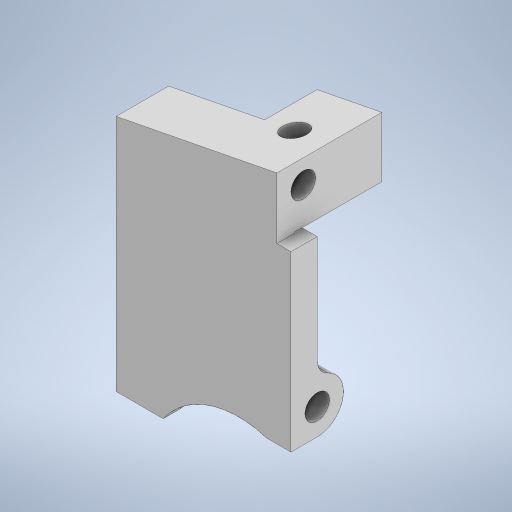
# Autodesk Inventor part: scianka_prawa
Saved by Autodesk Inventor 2023.5 (Build 275446000, 446)
## iProperties
Created: 2025-03-26
Part Number: scianka_prawa
Material: Ogólny
Document SubType Name: Modeling
Designer: kamil
Density: 1 g/cm^3
Appearance: Domyślna
Author: kamil
Autodesk Inventor part; units mm, degrees
ref_plane "YZ Plane" through (0, 0, 0) normal (1, 0, 0) x (0, 1, 0)
ref_plane "XZ Plane" through (0, 0, 0) normal (0, 1, 0) x (-1, 0, 0)
ref_plane "XY Plane" through (0, 0, 0) normal (0, 0, 1) x (1, 0, 0)
sketch "Szkic1" plane through (0, 0, 0) normal (0, 0, 1) x (1, 0, 0)
  line L0 (-34.4275, 20.8419) -> (2, 27.9622) projected
  line L1 (-2, 0) -> (-2, 27.1803) projected
  arc A0 (-16.6168, -4) -> (-14.1644, -18.5) centre (-8, -10) ccw projected
  circle A1 centre (-8, -10) radius 10.5
  line L2 (-2, 0) -> (-4.7984, 0)
  line L3 (-16.6168, -4) -> (-22, -4) projected
  line L4 (-22, 22.4466) -> (-22, 0.5) projected
  line L5 (-22, -4) -> (-22, 0.5)
  line L6 (-22, 22.4466) -> (-22, 23.271)
  point P0 (0, 0)
  constraints: 6 end point, 2 vertical, 1 coincident, 1 horizontal, 1 point on line, 4 other
extrude "Wyciągnięcie proste1" add sketch "Szkic1" against normal blind 2 contours L0 L1 L2 A1 L3 L5 L4 L6
sketch "Szkic2" plane through (-22, -4, 0) normal (-1, 0, 0) x (0, 0, 1)
  circle A0 centre (-2.5, 5.5) radius 1.3 projected
  line L0 (0, 27.271) -> (0, 0) projected
  circle A1 centre (-2.5, 5.5) radius 2.5
  line L1 (0, 27.271) -> (0, 0) projected
  line L2 (0, 27.271) -> (-2, 27.271) projected
  line L3 (-2, 0) -> (-2, 27.271) projected
  line L4 (0, 0) -> (-2, 0) projected
  line L5 (-2, 0) -> (-4.6176, 4.1711)
  line L6 (-2, 0) -> (-2, 27.271) projected
  line L7 (-2, 11) -> (-4.6176, 6.8289)
  point P0 (0, 4)
  constraints: 4 end point, 3 tangent, 2 point on circle, 1 centre point, 1 coincident, 1 point on line, 1 vertical alignment
extrude "Wyciągnięcie proste2" add sketch "Szkic2" against normal blind 5 contours L3 A0 | A0 L3 A1 | A1 L7 L3 | L3 L5 A1 picked at (-2.9631, 5.7248) picked at (-2.3031, 3.4223)
sketch "Szkic3" plane through (0, 0, -2) normal (0, 0, -1) x (-1, 0, 0)
  line L0 (2.5, 6.5) -> (19.5, 6.5) projected
  line L1 (2.5, 19.5) -> (2.5, 6.5) projected
  line L2 (19.5, 19.5) -> (2.5, 19.5) projected
  line L3 (19.5, 6.5) -> (19.5, 19.5) projected
  line L4 (2.5, 20) -> (19.5, 20) projected
  line L5 (17, 7) -> (22, 7) projected
  line L6 (22, 7) -> (22, 23.271) projected
  line L7 (22, 23.271) -> (2, 27.1803) projected
  line L8 (2, 27.1803) -> (2, 0) projected
  line L9 (2, 0) -> (4.7984, 0) projected
  arc A0 (16.6168, -4) -> (4.7984, 0) centre (8, -10) ccw projected
  line L10 (16.6168, -4) -> (17, -4) projected
  line L11 (17, -4) -> (17, 7) projected
  line L12 (19.5, 20) -> (22, 20)
  line L13 (22, 7) -> (22, 23.271) projected
  line L14 (2.5, 20) -> (2, 20)
  line L15 (2, 0) -> (2, 27.1803) projected
  point P0 (0, 0)
  constraints: 4 end point, 3 point on line, 1 perpendicular
extrude "Wyciągnięcie proste3" add sketch "Szkic3" along normal blind 4 contours L12 L4 L14 L8 L7 L6
sketch "Szkic4" plane through (0, 0, -6) normal (0, 0, -1) x (-1, 0, 0)
  line L0 (2, 20) -> (22, 20) projected
  line L1 (22, 20) -> (22, 23.271) projected
  line L2 (22, 23.271) -> (2, 27.1803) projected
  line L3 (2, 27.1803) -> (2, 20) projected
  line L4 (12.0145, 25.2228) -> (12.0145, 21) projected
  line L5 (12.0145, 21) -> (12, 20)
  line L6 (22, 20) -> (2, 20) projected
  point P0 (0, 0)
  constraints: 2 end point, 1 midpoint
extrude "Wyciągnięcie proste4" add sketch "Szkic4" along normal blind 6 contours L3 L2 L4 L5 L0
sketch "Szkic5" plane through (-12.0145, 21, -6) normal (-1, 0, 0) x (0, 0, 1)
  line L0 (0, 4.2228) -> (0, 0) projected
  line L1 (0, 4.2228) -> (-6, 4.2228) projected
  line L2 (-6, 0) -> (-6, 4.2228) projected
  line L3 (0, 0) -> (-6, 0) projected
  line L4 (0, 0) -> (-6, 0) projected
  line L5 (0, 0) -> (0, -1) projected
  line L6 (0, 0) -> (-6, 0) projected
  line L7 (-6, -1) -> (-6, 0) projected
  line L8 (0, -1) -> (-6, -1) projected
  line L9 (-6, -1) -> (0, -1)
  line L10 (0, -1) -> (0, 13.1761)
  line L11 (0, 13.1761) -> (-6, 13.1761)
  line L12 (-6, 13.1761) -> (-6, -1)
  point P0 (6, -21)
  constraints: 8 end point, 2 parallel, 1 horizontal, 1 perpendicular
extrude "Wyciągnięcie proste5" cut sketch "Szkic5" against normal blind 1
sketch "Szkic6" plane through (-22, 23.271, 0) normal (-0.1918332, 0.9814276, 0) x (0.9814276, 0.1918332, 0)
  line L0 (11.1933, 12) -> (11.1933, 6) projected
  line L1 (0, 6) -> (11.1933, 6) projected
  line L2 (0, 0) -> (0, 6) projected
  line L3 (20.3785, 0) -> (0, 0) projected
  line L4 (20.3785, 0) -> (20.3785, 12) projected
  line L5 (11.1933, 12) -> (20.3785, 12) projected
  point P0 (17.1273, 0)
  point P1 (14.6964, 6)
  point P2 (20.3785, 6)
  dimension "d10" = 3.503
  constraints: 1 horizontal alignment, 1 midpoint
  measures "d10" distance from line of point (14.696, 6) L0
hole "Otwór1" at (-7.5766, 26.0903, -6) direction (0.1918332, -0.9814276, 0) diameter 2.8 end through all
sketch "Szkic7" plane through (-2, 0, 0) normal (1, 0, 0) x (0, 0, -1)
  line L0 (0, 0) -> (0, 27.1803) projected
  line L1 (0, 0) -> (2, 0) projected
  line L2 (2, 20) -> (2, 0) projected
  line L3 (2, 20) -> (12, 20) projected
  line L4 (12, 27.1803) -> (12, 20) projected
  line L5 (0, 27.1803) -> (12, 27.1803) projected
  circle A0 centre (3, 3) radius 3
  circle A1 centre (3, 24.1803) radius 3
  line L6 (0, 0) -> (2, 0) projected
  line L7 (3, 0) -> (2, 0)
  line L8 (3, 6) -> (2, 6)
  dimension "d18" = 6
  dimension "d19" = 6
  constraints: 4 end point, 3 horizontal, 2 tangent, 1 centre point, 1 perpendicular, 1 point on line, 1 vertical, 3 other
  measures "d19" diameter of A1
extrude "Wyciągnięcie proste6" add sketch "Szkic7" against normal blind 3 contours L2 A0 L7 | A0 L2 | L2 L8 A0 picked at (2.9568, 3.7818)
sketch "Szkic8" plane through (-2, 0, 0) normal (1, 0, 0) x (0, 0, -1)
  arc A0 (3, 0) -> (3, 6) centre (3, 3) ccw projected
  line L0 (0, 0) -> (0, 27.1803) projected
  line L1 (0, 0) -> (3, 0) projected
  arc A1 (3, 0) -> (3, 6) centre (3, 3) ccw projected
  line L2 (3, 6) -> (2, 6) projected
  line L3 (2, 20) -> (2, 6) projected
  line L4 (2, 20) -> (12, 20) projected
  line L5 (12, 27.1803) -> (12, 20) projected
  line L6 (0, 27.1803) -> (12, 27.1803) projected
  circle A2 centre (3, 24.1803) radius 3
  point P0 (0, 0)
  dimension "d22" = 6
  constraints: 2 tangent, 1 centre point
  measures "d22" diameter of A2
hole "Otwór2" at (-2, 3, -3) at (-2, 24.1803, -3) direction (-1, 0, 0) diameter 2.8 depth 5 tip angle 118
sketch "Szkic9" plane through (-22, -4, 0) normal (-1, 0, 0) x (0, 0, 1)
  circle A0 centre (-2.5, 5.5) radius 1.3 projected
  point P0 (0, 4)
hole "Otwór3" at (-22, 1.5, -2.5) direction (1, 0, 0) diameter 2.3 depth 7 tip angle 118
sketch "Szkic10" plane through (0, 0, 0) normal (0, 0, 1) x (1, 0, 0)
  line L0 (-22, 23.271) -> (-22, -4) projected
  line L1 (-22, -4) -> (-16.6168, -4) projected
  arc A0 (-4.7984, 0) -> (-16.6168, -4) centre (-8, -10) ccw projected
  line L2 (-4.7984, 0) -> (-2, 0) projected
  line L3 (-2, 0) -> (-2, 27.1803) projected
  line L4 (-2, 27.1803) -> (-22, 23.271) projected
  line L5 (-2, 20.8676) -> (-3.6, 20.8676) projected
  line L6 (-2, 20.8676) -> (-2, 25.8676) projected
  line L7 (-3.6, 25.8676) -> (-2, 25.8676) projected
  line L8 (-3.6, 20.8676) -> (-3.6, 25.8676) projected
  line L9 (-2, 0) -> (-2, 27.1803) projected
  line L10 (-2, 27.1803) -> (-3.6, 27.1803)
  line L11 (-3.6, 27.1803) -> (-3.6, 19.8676)
  line L12 (-3.6, 19.8676) -> (-2, 19.8676)
  line L13 (-2, 19.8676) -> (-2, 27.1803)
  line L14 (-2, 19.8676) -> (-3.6, 19.8676) projected
  point P0 (0, 0)
  constraints: 8 end point, 2 collinear, 2 parallel, 1 horizontal, 1 perpendicular
extrude "Wyciągnięcie proste7" cut sketch "Szkic10" against normal through all contours L11 L10 L4 | L4 L3 L7 L11 | L7 L3 L5 L8 | L5 L3 L12 L11
sketch "Szkic11" plane through (-2, 3, -3) normal (1, 0, 0) x (0, 0, -1)
  line L0 (-1, 16.8676) -> (-3, 16.8676) projected
  line L1 (-3, -3) -> (-3, 16.8676) projected
  line L2 (-3, -3) -> (0, -3) projected
  arc A0 (0, -3) -> (0, 3) centre (0, 0) ccw projected
  line L3 (0, 3) -> (-1, 3) projected
  line L4 (-1, 16.8676) -> (-1, 3) projected
  circle A1 centre (0, 0) radius 1.4 projected
  line L5 (-1, 16.8676) -> (0, 16.8676)
  line L6 (0, 16.8676) -> (0, 3)
  line L7 (0, 3) -> (-1, 3)
  line L8 (-1, 3) -> (-1, 16.8676)
  point P0 (-3, -3)
  dimension "d40" = 1
  constraints: 8 end point, 2 parallel, 1 horizontal, 1 perpendicular
  measures "d40" distance between parallel lines of L6 L4
extrude "Wyciągnięcie proste8" add sketch "Szkic11" against normal up to surface (3 mm away) contours L5 L6 L3 L4
fillet "Zaokrąglenie1" radius 2 1 edges at (-3.5, 6, -3)
